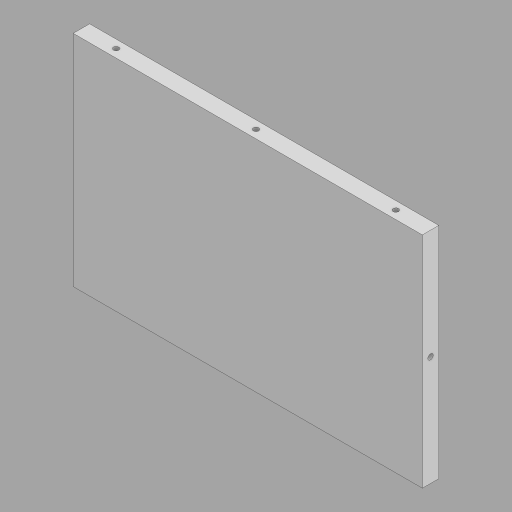
# Autodesk Inventor part: Lateral1-2
Saved by Autodesk Inventor 2023.2 (Build 272271030, 271C)
## iProperties
Created: 2023-04-15
Part Number: Lateral1-2
Material: Generic
Document SubType Name: Modeling
Designer: victo
Density: 1 g/cm^3
Appearance: Default
Author: victo
## iProperties of the stored document Lateral1-2_3DPrint.ipt
Created: 2023-05-16
Part Number: Lateral1-2_3DPrint
Material: Generic
Document SubType Name: Modeling
Designer: VICTOR
Density: 1 g/cm^3
Appearance: Default
Author: VICTOR
Autodesk Inventor part; units mm, degrees
ref_plane "YZ Plane" through (0, 0, 0) normal (1, 0, 0) x (0, 1, 0)
ref_plane "XZ Plane" through (0, 0, 0) normal (0, 1, 0) x (-1, 0, 0)
ref_plane "XY Plane" through (0, 0, 0) normal (0, 0, 1) x (1, 0, 0)
sketch "Sketch1" plane through (0, 0, 0) normal (0, 0, 1) x (1, 0, 0)
  line L0 (0, 0) -> (191, 0)
  line L1 (191, 0) -> (191, 120)
  line L2 (191, 120) -> (0, 120)
  line L3 (0, 120) -> (0, 0)
  dimension "d0" = 191
  dimension "d1" = 120
  constraints: 8 end point, 2 parallel, 1 horizontal, 1 perpendicular
  measures "d0" distance of L2.end L1.end
  measures "d1" distance of L1.end L0.end
extrude "Extrusion1" add sketch "Sketch1" along normal blind 9
sketch "Sketch2" plane through (0, 120, 0) normal (0, 1, 0) x (1, 0, 0)
  line L0 (191, 0) -> (0, 0) projected
  line L1 (0, 0) -> (0, -9) projected
  line L2 (191, -9) -> (0, -9) projected
  line L3 (191, 0) -> (191, -9) projected
  circle A0 centre (19, -4.5) radius 1.5
  circle A1 centre (95.5, -4.5) radius 1.5
  circle A2 centre (172, -4.5) radius 1.5
  point P0 (0, 0)
  dimension "d4" = 3
  dimension "d5" = 3
  dimension "d6" = 3
  dimension "d18" = 76.5
  constraints: 3 centre point
  measures "d4" diameter of A0
  measures "d5" diameter of A1
  measures "d6" diameter of A2
  measures "d18" distance of A1.centre A0.centre
extrude "Extrusion2" cut sketch "Sketch2" against normal blind 10 contours A0 | A1 | A2
sketch "Sketch3" plane through (0, 0, 0) normal (0, -1, 0) x (1, 0, 0)
  circle A0 centre (19, 4.5) radius 1.5 projected
  circle A1 centre (172, 4.5) radius 1.5 projected
  circle A2 centre (95.5, 4.5) radius 1.5
  line L0 (191, 0) -> (191, 9) projected
  point P0 (0, 0)
  dimension "d15" = 3
  dimension "d17" = 76.5
  constraints: 1 centre point
  measures "d15" diameter of A2
  measures "d17" distance of A0.centre A2.centre
extrude "Extrusion3" cut sketch "Sketch3" against normal blind 10
sketch "Sketch4" plane through (191, 0, 0) normal (1, 0, 0) x (0, 0, -1)
  line L0 (0, 0) -> (0, 120) projected
  line L1 (0, 120) -> (-9, 120) projected
  line L2 (-9, 0) -> (-9, 120) projected
  line L3 (0, 0) -> (-9, 0) projected
  circle A0 centre (-4.5, 60) radius 1.5
  point P0 (0, 0)
  dimension "d11" = 3
  constraints: 1 centre point
  measures "d11" diameter of A0
extrude "Extrusion4" cut sketch "Sketch4" against normal blind 10 contours A0
body "Solid1"
